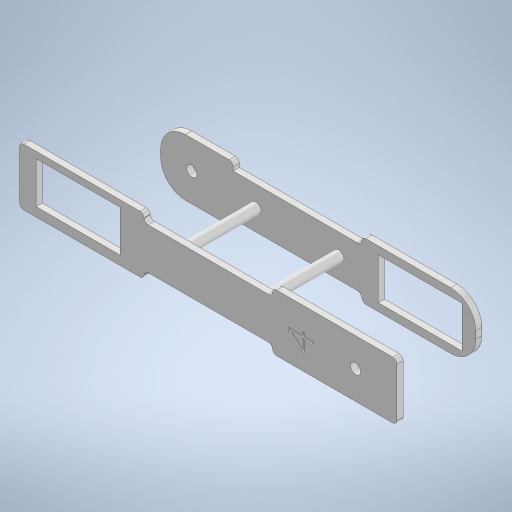
# Autodesk Inventor part: Pieza_eslabon_4
Saved by Autodesk Inventor 2023 (Build 270158000, 158)
## iProperties
Created: 2024-09-27
Part Number: Pieza_eslabon_4
Material: Genérico
Document SubType Name: Sheet Metal
Designer: sebas
Density: 1 g/cm^3
Sheet Metal Rule: Por defecto_mm
Appearance: Valor por defecto
Author: sebas
Autodesk Inventor part; units mm, degrees
ref_plane "YZ Plane" through (0, 0, 0) normal (1, 0, 0) x (0, 1, 0)
sketch "Boceto1" plane through (0, 0, 0) normal (0, 0, 1) x (1, 0, 0)
  line L0 (-91, 11.75) -> (-91, -11.75)
  line L1 (-89, -13.75) -> (-33, -13.75)
  line L2 (-31, -11.75) -> (-31, -12)
  line L3 (-29, -10) -> (29, -10)
  line L4 (31, -12) -> (31, -11.75)
  line L5 (33, -13.75) -> (89, -13.75)
  line L6 (91, -11.75) -> (91, 11.75)
  line L7 (89, 13.75) -> (33, 13.75)
  line L8 (31, 11.75) -> (31, 12)
  line L9 (29, 10) -> (-29, 10)
  line L10 (-31, 12) -> (-31, 11.75)
  line L11 (-33, 13.75) -> (-89, 13.75)
  line L12 (0, 0) -> (0, 52.9432) construction
  line L13 (0, 0) -> (-66, 0) construction
  arc A0 (-89, 13.75) -> (-91, 11.75) centre (-89, 11.75) ccw
  arc A1 (-91, -11.75) -> (-89, -13.75) centre (-89, -11.75) ccw
  arc A2 (-33, -13.75) -> (-31, -11.75) centre (-33, -11.75) ccw
  arc A3 (-29, -10) -> (-31, -12) centre (-29, -12) ccw
  arc A4 (-31, 12) -> (-29, 10) centre (-29, 12) ccw
  arc A5 (-31, 11.75) -> (-33, 13.75) centre (-33, 11.75) ccw
  arc A6 (29, 10) -> (31, 12) centre (29, 12) ccw
  arc A7 (33, 13.75) -> (31, 11.75) centre (33, 11.75) ccw
  arc A8 (31, -12) -> (29, -10) centre (29, -12) ccw
  arc A9 (31, -11.75) -> (33, -13.75) centre (33, -11.75) ccw
  arc A10 (89, -13.75) -> (91, -11.75) centre (89, -11.75) ccw
  arc A11 (91, 11.75) -> (89, 13.75) centre (89, 11.75) ccw
  point P0 (-91, 13.75)
  point P1 (-91, -13.75)
  point P2 (-31, -13.75)
  point P3 (91, -13.75)
  point P4 (91, 13.75)
  point P5 (31, 13.75)
  point P6 (31, 10)
  point P7 (-31, 10)
  point P8 (-31, 13.75)
  dimension "d0" = 182
  dimension "d1" = 60
  dimension "d3" = 27.5
  dimension "d4" = 20
  dimension "d5" = 2
  dimension "d6" = 27.5
  dimension "d7" = 2
  constraints: 28 end point, 24 point on circle, 24 tangent, 22 point on line, 12 centre point, 10 equal radius, 8 perpendicular, 3 horizontal, 1 collinear, 1 vertical, 4 other
  measures "d0" distance between parallel lines of L6 L0
  measures "d1" distance of point (-91, -13.75) point (-31, -13.75)
  measures "d3" distance of point (-91, 13.75) point (-91, -13.75)
  measures "d4" distance between parallel lines of L3 L9
  measures "d5" radius of A0
  measures "d6" distance of point (91, -13.75) point (91, 13.75)
  measures "d7" radius of A6
extrude "Extrusión1" add sketch "Boceto1" along normal blind 3
sketch "Boceto2" plane through (0, 0, 3) normal (0, 0, 1) x (1, 0, 0)
  circle A0 centre (-20, 0) radius 2.5
  circle A1 centre (20, 0) radius 2.5
  line L0 (0, 0) -> (0, 32) construction
  dimension "d10" = 5
  dimension "d11" = 5
  dimension "d12" = 40
  constraints: 2 centre point, 2 end point, 1 symmetric about line, 1 vertical
  measures "d10" diameter of A0
  measures "d11" diameter of A1
  measures "d12" distance of A1.centre A0.centre
extrude "Extrusión2" cut sketch "Boceto2" against normal blind 3
ref_plane "Plano de trabajo1" through (0, 0, -40) normal (0, 0, -1) x (-1, 0, 0)
sketch "Boceto3" plane through (0, 0, -40) normal (0, 0, -1) x (-1, 0, 0)
  line L0 (-86, 1.75) -> (-86, -1.75)
  line L1 (-74, -13.75) -> (-33, -13.75)
  line L2 (-31, -11.75) -> (-31, -12)
  line L3 (-29, -10) -> (29, -10)
  line L4 (31, -12) -> (31, -11.75)
  line L5 (33, -13.75) -> (54, -13.75)
  line L6 (66, -1.75) -> (66, 1.75)
  line L7 (54, 13.75) -> (33, 13.75)
  line L8 (31, 11.75) -> (31, 10)
  line L9 (31, 10) -> (-29, 10)
  line L10 (-31, 12) -> (-31, 11.75)
  line L11 (-33, 13.75) -> (-74, 13.75)
  line L12 (0, 0) -> (0, 26) construction
  line L13 (0, 0) -> (49, 0) construction
  arc A0 (-74, 13.75) -> (-86, 1.75) centre (-74, 1.75) ccw
  arc A1 (-86, -1.75) -> (-74, -13.75) centre (-74, -1.75) ccw
  arc A2 (66, 1.75) -> (54, 13.75) centre (54, 1.75) ccw
  arc A3 (54, -13.75) -> (66, -1.75) centre (54, -1.75) ccw
  arc A4 (-31, 11.75) -> (-33, 13.75) centre (-33, 11.75) ccw
  arc A5 (-31, 12) -> (-29, 10) centre (-29, 12) ccw
  arc A6 (-29, -10) -> (-31, -12) centre (-29, -12) ccw
  arc A7 (-33, -13.75) -> (-31, -11.75) centre (-33, -11.75) ccw
  arc A8 (33, 13.75) -> (31, 11.75) centre (33, 11.75) ccw
  arc A9 (31, -11.75) -> (33, -13.75) centre (33, -11.75) ccw
  arc A10 (31, -12) -> (29, -10) centre (29, -12) ccw
  point P0 (-86, 13.75)
  point P1 (-86, -13.75)
  point P2 (66, -13.75)
  point P3 (66, 13.75)
  point P4 (31, 13.75)
  point P5 (-31, 10)
  point P6 (-31, 13.75)
  dimension "d16" = 27.5
  dimension "d17" = 27.5
  dimension "d18" = 152
  dimension "d19" = 55
  dimension "d21" = 62
  dimension "d22" = 20
  dimension "d23" = 12
  dimension "d24" = 2
  constraints: 28 end point, 22 point on circle, 22 tangent, 16 point on line, 11 centre point, 9 equal radius, 8 perpendicular, 3 vertical, 2 horizontal, 1 parallel, 4 other
  measures "d16" distance of point (66, -13.75) point (66, 13.75)
  measures "d17" distance of point (-86, 13.75) point (-86, -13.75)
  measures "d18" distance between parallel lines of L6 L0
  measures "d19" distance of point (-31, 13.75) point (-86, 13.75)
  measures "d21" distance of L8.end point (-31, 10)
  measures "d22" distance between parallel lines of L3 L9
  measures "d23" radius of A0
  measures "d24" radius of A4
extrude "Extrusión3" add sketch "Boceto3" along normal blind 3
sketch "Boceto4" plane through (0, 0, -43) normal (0, 0, -1) x (-1, 0, 0)
  circle A0 centre (-20, 0) radius 2.5 projected
  circle A1 centre (20, 0) radius 2.5 projected
  point P0 (0, 0)
extrude "Extrusión4" cut sketch "Boceto4" against normal blind 3
sketch "Boceto5" plane through (0, 0, 3) normal (0, 0, 1) x (1, 0, 0)
  line L0 (-51, 21) -> (-51, -25) construction
  line L1 (71, 20) -> (71, -24) construction
  line L2 (31, -12) -> (31, -11.75) projected
  circle A0 centre (-51, 0) radius 2.5
  circle A1 centre (71, 0) radius 2.5
  line L3 (-91, 11.75) -> (-91, -11.75) projected
  point P0 (31, -11.875)
  dimension "d32" = 40
  dimension "d34" = 5
  dimension "d35" = 5
  dimension "d46" = 40
  constraints: 4 end point, 2 centre point, 2 point on line, 2 vertical, 1 midpoint
  measures "d32" distance from line of L1 point (31, -11.875)
  measures "d34" diameter of A0
  measures "d35" diameter of A1
  measures "d46" distance between parallel lines of L3 L0
extrude "Extrusión5" cut sketch "Boceto5" against normal up to surface (46 mm away)
sketch "Boceto6" plane through (0, 0, -43) normal (0, 0, -1) x (-1, 0, 0)
  circle A0 centre (51, 0) radius 2.5
  line L0 (31, 11.75) -> (31, 10) projected
  point P0 (0, 0)
  point P1 (31, 10.875)
  dimension "d38" = 5
  dimension "d39" = 20
  constraints: 1 centre point, 1 midpoint
  measures "d38" diameter of A0
  measures "d39" horizontal distance of point (31, 10.875) A0.centre
extrude "Extrusión6" cut sketch "Boceto6" against normal blind 3
ref_plane "Plano de trabajo2" through (0, 0, -20) normal (0, 0, -1) x (-1, 0, 0)
sketch "Boceto7" plane through (0, 0, -20) normal (0, 0, -1) x (-1, 0, 0)
  circle A0 centre (20, 0) radius 2.5 projected
  circle A1 centre (-20, 0) radius 2.5 projected
  point P0 (0, 0)
extrude "Extrusión7" add sketch "Boceto7" along normal mid plane 46
sketch "Boceto8" plane through (0, 0, 3) normal (0, 0, 1) x (1, 0, 0)
  line L0 (38.7008, -6.0818) -> (38.7008, 17.3731) construction
  line L1 (38.7008, 17.3731) -> (57.2312, 17.3731) construction
  line L2 (57.2312, 17.3731) -> (57.2312, -6.0818) construction
  line L3 (57.2312, -6.0818) -> (38.7008, -6.0818) construction
  line L4 (46.5776, 2.5146) -> (46.5776, 1.0851)
  line L5 (46.5776, 1.0851) -> (50.7008, 1.0851)
  line L6 (50.7008, 1.0851) -> (50.7008, -0.461)
  line L7 (50.7008, -0.461) -> (46.5776, -0.461)
  line L8 (46.5776, -0.461) -> (46.5776, -5.7609)
  line L9 (46.5776, -5.7609) -> (44.8855, -5.7609)
  line L10 (44.8855, -5.7609) -> (38.7008, -0.393)
  line L11 (38.7008, -0.393) -> (38.7008, 1.0851)
  line L12 (38.7008, 1.0851) -> (45.2842, 1.0851)
  line L13 (45.2842, 1.0851) -> (45.2842, 2.5146)
  line L14 (45.2842, 2.5146) -> (46.5776, 2.5146)
  line L15 (45.2842, -0.461) -> (40.597, -0.461)
  line L16 (40.597, -0.461) -> (45.2842, -4.4967)
  line L17 (45.2842, -4.4967) -> (45.2842, -0.461)
  point P0 (0, 0)
  constraints: 2 other
extrude "Extrusión8" cut sketch "Boceto8" against normal blind 0.5
sketch "Boceto9" plane through (0, 0, 3) normal (0, 0, 1) x (1, 0, 0)
  line L0 (-83, 10.6047) -> (-42.6, 10.6047)
  line L1 (-42.6, 10.6047) -> (-42.6, -9.3953)
  line L2 (-42.6, -9.3953) -> (-83, -9.3953)
  line L3 (-83, -9.3953) -> (-83, 10.6047)
  line L4 (-91, 11.75) -> (-91, -11.75) construction
  point P0 (0, 0)
  dimension "d47" = 40.4
  dimension "d48" = 20
  dimension "d49" = 8
  constraints: 8 end point, 2 parallel, 1 horizontal, 1 perpendicular
  measures "d47" distance between parallel lines of L3 L1
  measures "d48" distance between parallel lines of L2 L0
  measures "d49" distance between parallel lines of L4 L3
extrude "Extrusión9" cut sketch "Boceto9" against normal up to surface (3 mm away)
sketch "Boceto10" plane through (0, 0, -43) normal (0, 0, -1) x (-1, 0, 0)
  line L0 (-79.4, 10) -> (-39, 10)
  line L1 (-39, 10) -> (-39, -10)
  line L2 (-39, -10) -> (-79.4, -10)
  line L3 (-79.4, -10) -> (-79.4, 10)
  line L4 (-71, 0) -> (-43, 0) construction
  line L5 (-31, 12) -> (-31, 11.75) projected
  point P0 (0, 0)
  point P1 (-31, 11.875)
  dimension "d52" = 40.4
  dimension "d53" = 20
  dimension "d54" = 8
  constraints: 10 end point, 2 parallel, 1 horizontal, 1 midpoint, 1 perpendicular, 1 other
  measures "d52" distance of L1.end L2.end
  measures "d53" distance of L0.end L1.end
  measures "d54" distance from line of point (-31, 11.875) L1
extrude "Extrusión10" cut sketch "Boceto10" against normal blind 3
equation "\"Radio_pliegue\" = Grosor"
equation "\"Anchura_desahogo_plegado\" = Grosor"
equation "\"Profundidad_desahogo_plegado\" = 0.5 * Grosor"
equation "\"Tamaño_destalonado\" = 4 * Grosor"
equation "\"Remanente_mínimo\" = 2 * Grosor"
equation "\"Radiodetransición\" = Radio_pliegue"
equation "\"Tamaño_de_radio_de_Jacobi\" = Radio_pliegue"
equation "\"TamañoSeparación\" = Grosor"
equation "\"Grosor\" = 0.5"
